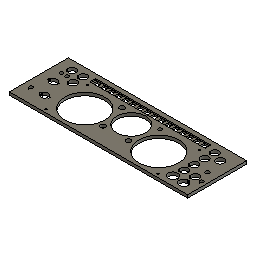
unimog dash old style (Autodesk Fusion 360 design; units mm, degrees)
part number: 2026-06-18-12-45-24-392
Autodesk Fusion 360 part; units mm, degrees
sketch "Sketch1" plane through (0, 0, 0) normal (0, 1, 0) x (1, 0, 0)
  line L0 (0, 0) -> (650, 0)
  line L1 (650, 0) -> (650, 215)
  line L2 (650, 215) -> (0, 215)
  line L3 (0, 215) -> (0, 0)
  circle A0 centre (47.25, 182) radius 14
  circle A1 centre (87.25, 182) radius 14
  circle A2 centre (36, 154.5) radius 6
  circle A3 centre (56, 154.5) radius 6
  circle A4 centre (87.25, 145) radius 14
  circle A5 centre (47.25, 113.3) radius 13.2
  circle A6 centre (75.25, 53.75) radius 13.2
  circle A7 centre (25.25, 53.75) radius 6.25
  circle A8 centre (121.1645, 163.2) radius 3.4
  circle A9 centre (25.0509, 44.2521) radius 1.25
  circle A10 centre (121.1645, 12.4) radius 3.4
  circle A11 centre (190.3639, 84.625) radius 72.625
  circle A12 centre (255.4078, 155.4015) radius 9
  circle A13 centre (325.3694, 119.25) radius 52.75
  circle A14 centre (392.7247, 157.0764) radius 6
  circle A15 centre (460.375, 84.625) radius 72.625
  circle A16 centre (278.8118, 62.6996) radius 9
  circle A17 centre (371.927, 62.6996) radius 9
  circle A18 centre (529.5743, 163.2) radius 3.4
  circle A19 centre (529.5743, 12.4) radius 3.4
  circle A20 centre (567.25, 182) radius 14
  circle A21 centre (567.25, 145) radius 14
  circle A22 centre (567.25, 108) radius 14
  circle A23 centre (567.25, 71) radius 14
  circle A24 centre (563.125, 33.275) radius 16.875
  circle A25 centre (607.25, 71) radius 14
  circle A26 centre (605.25, 30) radius 16
  circle A27 centre (633.75, 68.25) radius 6.25
  circle A28 centre (615.85, 107.15) radius 7.15
  circle A29 centre (602.5, 166.5) radius 14.5
  line L4 (567.25, 71) -> (567.25, 182) construction
  line L5 (567.25, 71) -> (607.25, 71) construction
  line L6 (529.5743, 12.4) -> (529.5743, 163.2) construction
  line L7 (594.9763, 67.5652) -> (603.8152, 58.7263) construction
  line L8 (607.25, 71) -> (597.3539, 61.1039) construction
  line L9 (607.25, 71) -> (621.2468, 71) construction
  line L10 (594.9763, 67.5652) -> (592.6482, 65.2371) construction
  line L11 (592.6482, 65.2371) -> (601.4871, 56.3982)
  line L12 (601.4871, 56.3982) -> (602.8112, 57.7223)
  line L13 (607.25, 71) -> (617.1495, 80.8995) construction
  line L14 (593.9723, 66.5612) -> (592.6482, 65.2371)
  line L15 (603.8152, 58.7263) -> (601.4871, 56.3982) construction
  line L16 (605.1938, 75.6264) -> (595.1802, 65.6128) construction
  line L17 (600.0149, 75.127) -> (608.8537, 66.2882) construction
  line L18 (608.8537, 66.2882) -> (601.6878, 59.1222) construction
  line L19 (592.8489, 67.9611) -> (601.6878, 59.1222)
  line L20 (600.0149, 75.127) -> (592.8489, 67.9611) construction
  line L21 (567.25, 71) -> (557.3505, 61.1005) construction
  line L22 (560.5418, 73.1307) -> (569.3807, 64.2918) construction
  line L23 (569.3807, 64.2918) -> (561.4871, 56.3982) construction
  line L24 (552.6482, 65.2371) -> (561.4871, 56.3982)
  line L25 (560.5418, 73.1307) -> (552.6482, 65.2371) construction
  line L26 (567.25, 108) -> (557.0677, 97.8177) construction
  line L27 (556.1832, 105.7721) -> (565.0221, 96.9332) construction
  line L28 (565.0221, 96.9332) -> (561.4871, 93.3982) construction
  line L29 (552.6482, 102.2371) -> (561.4871, 93.3982)
  line L30 (556.1832, 105.7721) -> (552.6482, 102.2371) construction
  line L31 (567.25, 145) -> (557.3539, 135.1039) construction
  line L32 (555.9409, 142.5297) -> (564.7797, 133.6909) construction
  line L33 (564.7797, 133.6909) -> (561.4871, 130.3982) construction
  line L34 (552.6482, 139.2371) -> (561.4871, 130.3982)
  line L35 (555.9409, 142.5297) -> (552.6482, 139.2371) construction
  line L36 (567.25, 182) -> (557.3505, 172.1005) construction
  line L37 (552.8238, 176.4127) -> (561.6627, 167.5738) construction
  line L38 (561.6627, 167.5738) -> (561.4871, 167.3982) construction
  line L39 (552.6482, 176.2371) -> (561.4871, 167.3982)
  line L40 (552.8238, 176.4127) -> (552.6482, 176.2371) construction
  line L41 (552.6482, 176.2371) -> (552.736, 176.3249)
  line L42 (552.736, 176.3249) -> (553.9723, 177.5612)
  line L43 (561.4871, 167.3982) -> (562.8112, 168.7223)
  line L44 (552.6482, 139.2371) -> (553.9723, 140.5612)
  line L45 (561.4871, 130.3982) -> (562.8112, 131.7223)
  line L46 (552.6482, 65.2371) -> (553.9723, 66.5612)
  line L47 (561.4871, 56.3982) -> (562.8112, 57.7223)
  line L48 (561.4871, 93.3982) -> (562.8112, 94.7223)
  line L49 (552.6482, 102.2371) -> (553.9723, 103.5612)
  line L50 (371.927, 62.6996) -> (278.8118, 62.6996) construction
  line L51 (460.375, 84.625) -> (190.3639, 84.625) construction
  line L52 (121.1645, 12.4) -> (529.5743, 12.4) construction
  line L53 (121.1645, 12.4) -> (121.1645, 163.2) construction
  line L54 (121.1645, 163.2) -> (529.5743, 163.2) construction
  line L55 (605.25, 14) -> (605.25, 30) construction
  line L56 (605.25, 30) -> (605.25, 46) construction
  line L57 (546.25, 33.275) -> (563.125, 33.275) construction
  line L58 (563.125, 33.275) -> (580, 33.275) construction
  line L59 (602, 48) -> (608.5, 48)
  line L60 (608.5, 48) -> (608.5, 43.3355)
  line L61 (608.5, 43.3355) -> (602, 43.3355)
  line L62 (602, 43.3355) -> (602, 48)
  line L63 (578.0171, 36.025) -> (580.75, 36.025)
  line L64 (580.75, 36.025) -> (580.75, 30.525)
  line L65 (580.75, 30.525) -> (578.0171, 30.525)
  line L66 (578.0171, 30.525) -> (578.0171, 36.025)
  circle A30 centre (633.75, 58.75) radius 1.25
  line L67 (633.75, 68.25) -> (633.75, 58.75) construction
  line L68 (87.25, 145) -> (77.3505, 135.1005) construction
  line L69 (87.25, 182) -> (77.3505, 172.1005) construction
  line L70 (47.25, 182) -> (37.3505, 172.1005) construction
  line L71 (87.25, 145) -> (87.25, 182) construction
  line L72 (87.25, 182) -> (47.25, 182) construction
  line L73 (36, 154.5) -> (56, 154.5) construction
  line L74 (567.25, 182) -> (87.25, 182) construction
  line L75 (557.3505, 61.1005) -> (557.0677, 60.8177) construction
  line L76 (557.3539, 135.1039) -> (550.2188, 127.9688) construction
  line L77 (32.3849, 176.5004) -> (41.2238, 167.6616)
  line L78 (32.3849, 176.5004) -> (33.8453, 177.9608)
  line L79 (41.2238, 167.6616) -> (42.4213, 168.8591)
  line L80 (87.25, 182) -> (76.9585, 171.7085) construction
  line L81 (72.6482, 176.2371) -> (74.0824, 177.2446)
  line L82 (81.4871, 167.3982) -> (82.8112, 168.7223)
  line L83 (87.25, 145) -> (77.0677, 134.8177) construction
  line L84 (72.6482, 139.2371) -> (73.9723, 140.5612)
  line L85 (72.6482, 139.2371) -> (81.4871, 130.3982)
  line L86 (81.4871, 130.3982) -> (82.8112, 131.7223)
  line L87 (72.6482, 176.2371) -> (81.4871, 167.3982)
  line L88 (76.9585, 171.7085) -> (77.0677, 171.8177) construction
  line L89 (30.5, 117.05) -> (64, 117.05)
  line L90 (64, 117.05) -> (64, 109.55)
  line L91 (64, 109.55) -> (30.5, 109.55)
  line L92 (30.5, 109.55) -> (30.5, 117.05)
  line L93 (47.25, 117.05) -> (47.25, 113.3) construction
  line L94 (47.25, 113.3) -> (30.5, 113.3) construction
  line L95 (92, 50) -> (58.5, 50)
  line L96 (75.25, 53.75) -> (58.5, 53.75) construction
  line L97 (75.25, 57.5) -> (75.25, 53.75) construction
  line L98 (58.5, 50) -> (58.5, 57.5)
  line L99 (58.5, 57.5) -> (92, 57.5)
  line L100 (92, 57.5) -> (92, 50)
  line L101 (47.25, 182) -> (47.25, 113.3) construction
  line L102 (75.25, 53.75) -> (25.25, 53.75) construction
  line L103 (115.3694, 199) -> (535.3694, 199)
  line L104 (535.3694, 199) -> (535.3694, 178.5)
  line L105 (535.3694, 178.5) -> (115.3694, 178.5)
  line L106 (115.3694, 178.5) -> (115.3694, 199)
  line L107 (325.3694, 119.25) -> (325.3694, 178.5) construction
  line L108 (122.3694, 198) -> (138.3694, 198)
  line L109 (138.3694, 198) -> (138.3694, 179.5)
  line L110 (138.3694, 179.5) -> (122.3694, 179.5)
  line L111 (122.3694, 179.5) -> (122.3694, 198)
  line L112 (115.3694, 188.75) -> (122.3694, 188.75)
  line L113 (148.3694, 179.5) -> (148.3694, 198)
  line L114 (148.3694, 198) -> (164.3694, 198)
  line L115 (164.3694, 198) -> (164.3694, 179.5)
  line L116 (164.3694, 179.5) -> (148.3694, 179.5)
  line L117 (174.3694, 179.5) -> (174.3694, 198)
  line L118 (174.3694, 198) -> (190.3694, 198)
  line L119 (190.3694, 198) -> (190.3694, 179.5)
  line L120 (190.3694, 179.5) -> (174.3694, 179.5)
  line L121 (200.3694, 179.5) -> (200.3694, 198)
  line L122 (200.3694, 198) -> (216.3694, 198)
  line L123 (216.3694, 198) -> (216.3694, 179.5)
  line L124 (216.3694, 179.5) -> (200.3694, 179.5)
  line L125 (226.3694, 179.5) -> (226.3694, 198)
  line L126 (226.3694, 198) -> (242.3694, 198)
  line L127 (242.3694, 198) -> (242.3694, 179.5)
  line L128 (242.3694, 179.5) -> (226.3694, 179.5)
  line L129 (252.3694, 179.5) -> (252.3694, 198)
  line L130 (252.3694, 198) -> (268.3694, 198)
  line L131 (268.3694, 198) -> (268.3694, 179.5)
  line L132 (268.3694, 179.5) -> (252.3694, 179.5)
  line L133 (278.3694, 179.5) -> (278.3694, 198)
  line L134 (278.3694, 198) -> (294.3694, 198)
  line L135 (294.3694, 198) -> (294.3694, 179.5)
  line L136 (294.3694, 179.5) -> (278.3694, 179.5)
  line L137 (304.3694, 179.5) -> (304.3694, 198)
  line L138 (304.3694, 198) -> (320.3694, 198)
  line L139 (320.3694, 198) -> (320.3694, 179.5)
  line L140 (320.3694, 179.5) -> (304.3694, 179.5)
  line L141 (330.3694, 179.5) -> (330.3694, 198)
  line L142 (330.3694, 198) -> (346.3694, 198)
  line L143 (346.3694, 198) -> (346.3694, 179.5)
  line L144 (346.3694, 179.5) -> (330.3694, 179.5)
  line L145 (356.3694, 179.5) -> (356.3694, 198)
  line L146 (356.3694, 198) -> (372.3694, 198)
  line L147 (372.3694, 198) -> (372.3694, 179.5)
  line L148 (372.3694, 179.5) -> (356.3694, 179.5)
  line L149 (382.3694, 179.5) -> (382.3694, 198)
  line L150 (382.3694, 198) -> (398.3694, 198)
  line L151 (398.3694, 198) -> (398.3694, 179.5)
  line L152 (398.3694, 179.5) -> (382.3694, 179.5)
  line L153 (408.3694, 179.5) -> (408.3694, 198)
  line L154 (408.3694, 198) -> (424.3694, 198)
  line L155 (424.3694, 198) -> (424.3694, 179.5)
  line L156 (424.3694, 179.5) -> (408.3694, 179.5)
  line L157 (434.3694, 179.5) -> (434.3694, 198)
  line L158 (434.3694, 198) -> (450.3694, 198)
  line L159 (450.3694, 198) -> (450.3694, 179.5)
  line L160 (450.3694, 179.5) -> (434.3694, 179.5)
  line L161 (460.3694, 179.5) -> (460.3694, 198)
  line L162 (460.3694, 198) -> (476.3694, 198)
  line L163 (476.3694, 198) -> (476.3694, 179.5)
  line L164 (476.3694, 179.5) -> (460.3694, 179.5)
  line L165 (486.3694, 179.5) -> (486.3694, 198)
  line L166 (486.3694, 198) -> (502.3694, 198)
  line L167 (502.3694, 198) -> (502.3694, 179.5)
  line L168 (502.3694, 179.5) -> (486.3694, 179.5)
  line L169 (512.3694, 179.5) -> (512.3694, 198)
  line L170 (512.3694, 198) -> (528.3694, 198)
  line L171 (528.3694, 198) -> (528.3694, 179.5)
  line L172 (528.3694, 179.5) -> (512.3694, 179.5)
  point P0 (599.3958, 63.1458)
  point P1 (605.25, 43.3355)
  point P2 (578.0171, 33.275)
  point P3 (557.0677, 60.8177)
  point P4 (557.0677, 134.8177)
  point P5 (557.0677, 97.8177)
  point P6 (77.3505, 172.1005)
  point P7 (77.0677, 134.8177)
  point P8 (77.0677, 171.8177)
  point P9 (75.25, 57.5)
  point P10 (325.3694, 178.5)
  dimension "d1" = 650
  dimension "d2" = 215
  dimension "d3" = 32
  dimension "d4" = 14
  dimension "d5" = 28.75
  dimension "d6" = 12.5
  dimension "d7" = 10
  dimension "d8" = 62
  dimension "d9" = 28
  dimension "d10" = 28
  dimension "d11" = 28
  dimension "d12" = 28
  dimension "d13" = 28
  dimension "d14" = 33.75
  dimension "d15" = 16.4
  dimension "d16" = 70
  dimension "d17" = 6.8
  dimension "d19" = 9
  dimension "d20" = 28.75
  dimension "d21" = 57
  dimension "d22" = 12
  dimension "d23" = 9
  dimension "d24" = 9
  dimension "d25" = 9
  dimension "d26" = 19
  dimension "d27" = 29
  dimension "d28" = 33
  dimension "d29" = 34
  dimension "d30" = 14.3
  dimension "d31" = 27
  dimension "d32" = 100
  dimension "d33" = 6.8
  dimension "d34" = 144
  dimension "d35" = 145.25
  dimension "d36" = 145.25
  dimension "d37" = 12
  dimension "d38" = 117
  dimension "d39" = 12.5
  dimension "d40" = 135
  dimension "d41" = 28.4
  dimension "d42" = 12.5
  dimension "d43" = 12.5
  dimension "d44" = 12.5
  dimension "d45" = 12.5
  dimension "d46" = 12.5
  dimension "d47" = 66.5
  dimension "d48" = 105.5
  dimension "d49" = 14
  dimension "d50" = 12
  dimension "d51" = 18
  dimension "d52" = 18
  dimension "d53" = 18
  dimension "d54" = 9.5
  dimension "d55" = 11.5
  dimension "d56" = 11.5
  dimension "d57" = 9.5
  dimension "d58" = 14
  dimension "d59" = 6.8
  dimension "d62" = 24
  dimension "d63" = 408.4098
  dimension "d64" = 24
  dimension "d65" = 20.5
  dimension "d66" = 18.5
  dimension "d67" = 17
  dimension "d70" = 14.5
  dimension "d71" = 6.8
  dimension "d74" = 6.5
  dimension "d75" = 34
  dimension "d76" = 5.5
  dimension "d77" = 34.5
  dimension "d78" = 2.5
  dimension "d79" = 2
  dimension "d80" = 28
  dimension "d81" = 28
  dimension "d82" = 28
  dimension "d83" = 12
  dimension "d84" = 12
  dimension "d85" = 2.5
  dimension "d86" = 2
  dimension "d87" = 12.5
  dimension "d88" = 19
  dimension "d89" = 47.5
  dimension "d90" = 12
  dimension "d91" = 9
  dimension "d92" = 33.25
  dimension "d93" = 30
  dimension "d94" = 54.5
  dimension "d95" = 8
  dimension "d96" = 28.4
  dimension "d98" = 28.4
  dimension "d99" = 28.4
  dimension "d100" = 12.5
  dimension "d101" = 28.4
  dimension "d102" = 12.5
  dimension "d103" = 12.5
  dimension "d104" = 28.4
  dimension "d105" = 28.4
  dimension "d106" = 26.4
  dimension "d107" = 26.4
  dimension "d108" = 33.5
  dimension "d110" = 33.5
  dimension "d112" = 7.5
  dimension "d113" = 3.75
  dimension "d114" = 27
  dimension "d115" = 41.5
  dimension "d116" = 20.5
  dimension "d117" = 420
  dimension "d118" = 6.5
  dimension "d119" = 16
  dimension "d120" = 18.5
  dimension "d121" = 7
  dimension "d124" = 26
  dimension "d125" = 0
  dimension "d126" = 7
  constraint horizontal L0
  constraint vertical L1
  constraint horizontal L2
  constraint vertical L3
  constraint coincident L0.start L3.end
  constraint coincident A23.centre L4.start
  constraint coincident A20.centre L4.end
  constraint coincident A21.centre L4
  constraint coincident A22.centre L4
  constraint vertical L4
  constraint coincident A25.centre L5.end
  constraint horizontal L5
  constraint coincident A19.centre L6.start
  constraint coincident A18.centre L6.end
  constraint vertical L6
  constraint horizontal L9
  constraint perpendicular L7 L8
  constraint midpoint L7 P0
  constraint coincident L8 P0
  constraint perpendicular L7 L10
  constraint perpendicular L10 L11
  constraint parallel L10 L12
  constraint collinear L8 L13
  constraint coincident A25 L13.end
  constraint coincident A25 L14.start
  constraint coincident L10 L14.start
  constraint perpendicular L11 L14
  constraint coincident A25 L12.end
  constraint perpendicular L11 L15
  constraint perpendicular L16 L17
  constraint perpendicular L17 L20
  constraint perpendicular L19 L20
  constraint perpendicular L18 L19
  constraint perpendicular L21 L22
  constraint perpendicular L22 L25
  constraint perpendicular L24 L25
  constraint perpendicular L23 L24
  constraint perpendicular L26 L27
  constraint perpendicular L27 L30
  constraint perpendicular L29 L30
  constraint perpendicular L28 L29
  constraint perpendicular L31 L32
  constraint perpendicular L32 L35
  constraint perpendicular L34 L35
  constraint perpendicular L33 L34
  constraint perpendicular L36 L37
  constraint perpendicular L37 L40
  constraint perpendicular L39 L40
  constraint perpendicular L38 L39
  constraint midpoint L40 L41.end
  constraint coincident A20 L42.end
  constraint coincident L40 L42.end
  constraint coincident A20 L43.end
  constraint coincident L38 L43.end
  constraint coincident L35 L44.end
  constraint coincident A21 L44.end
  constraint coincident A21 L45.end
  constraint coincident L33 L45.end
  constraint coincident A23 L46.end
  constraint coincident L25 L46.end
  constraint coincident L23 L47.end
  constraint coincident A23 L47.end
  constraint coincident A22 L48.end
  constraint coincident L28 L48.end
  constraint coincident L30 L49.end
  constraint coincident A22 L49.end
  constraint coincident A17.centre L50.start
  constraint coincident A16.centre L50.end
  constraint horizontal L50
  constraint coincident A15.centre L51.start
  constraint coincident A11.centre L51.end
  constraint horizontal L51
  constraint coincident A10.centre L52.start
  constraint horizontal L52
  constraint coincident A8.centre L53.end
  constraint vertical L53
  constraint horizontal L54
  constraint coincident A26 L55.start
  constraint coincident A26.centre L55.end
  constraint coincident A26 L56.end
  constraint perpendicular L0 L56
  constraint collinear L55 L56
  constraint coincident A24 L57.start
  constraint coincident A24.centre L57.end
  constraint coincident A24 L58.end
  constraint parallel L57 L58
  constraint horizontal L58
  constraint horizontal L59
  constraint vertical L60
  constraint horizontal L61
  constraint vertical L62
  constraint midpoint L61 P1
  constraint coincident L56 P1
  constraint horizontal L63
  constraint vertical L64
  constraint horizontal L65
  constraint vertical L66
  constraint midpoint L66 P2
  constraint coincident L58 P2
  constraint coincident A27.centre L67.start
  constraint coincident A30.centre L67.end
  constraint vertical L67
  constraint coincident A4.centre L68.start
  constraint coincident A1.centre L69.start
  constraint coincident L70 A0.centre
  constraint horizontal L72
  constraint vertical L71
  constraint coincident A0.centre L70.start
  constraint coincident A2.centre L73.start
  constraint coincident A3.centre L73.end
  constraint horizontal L73
  constraint horizontal L74
  constraint coincident A23 L21.end
  constraint midpoint L24 P3
  constraint coincident P3 L75.end
  constraint perpendicular L24 L75
  constraint parallel L16 L21
  constraint parallel L8 L16
  constraint parallel L21 L26
  constraint parallel L26 L31
  constraint coincident A20 L36.end
  constraint perpendicular L32 L76
  constraint coincident A21.centre L31.start
  constraint midpoint L34 P4
  constraint coincident L76 P4
  constraint coincident A22.centre L26.start
  constraint coincident P5 L29
  constraint midpoint L29 P5
  constraint coincident P5 L26.end
  constraint coincident A1 P6
  constraint coincident A0 L70.end
  constraint coincident A4 L68.end
  constraint perpendicular L70 L77
  constraint coincident A0 L78.end
  constraint perpendicular L77 L78
  constraint coincident A0 L79.end
  constraint perpendicular L77 L79
  constraint coincident P6 L69.end
  constraint collinear L69 L80
  constraint coincident A1 L82.end
  constraint coincident A1 L81.end
  constraint perpendicular L83 L85
  constraint perpendicular L84 L85
  constraint perpendicular L85 L86
  constraint coincident P7 L85
  constraint parallel L68 L69
  constraint parallel L68 L83
  constraint midpoint L85 P7
  constraint coincident P7 L83.end
  constraint coincident A4 L84.end
  constraint coincident A4 L86.end
  constraint perpendicular L82 L87
  constraint midpoint L87 P8
  constraint parallel L69 L88
  constraint coincident P8 L88.end
  constraint parallel L70 L80
  constraint parallel L77 L87
  constraint horizontal L89
  constraint vertical L90
  constraint horizontal L91
  constraint vertical L92
  constraint midpoint L89 L93.start
  constraint coincident A5.centre L93.end
  constraint vertical L93
  constraint midpoint L92 L94.end
  constraint horizontal L94
  constraint vertical L100
  constraint horizontal L95
  constraint vertical L98
  constraint vertical L97
  constraint midpoint L96.end L98
  constraint horizontal L96
  constraint horizontal L99
  constraint coincident A6.centre L96.start
  constraint vertical L101
  constraint midpoint L99 P9
  constraint coincident P9 L97.start
  constraint coincident L98.end L99.start
  constraint coincident L99.end L100.start
  constraint coincident A7.centre L102.end
  constraint horizontal L102
  constraint horizontal L103
  constraint vertical L104
  constraint horizontal L105
  constraint vertical L106
  constraint midpoint L105 P10
  constraint coincident A13.centre L107.start
  constraint coincident P10 L107.end
  constraint vertical L107
  constraint horizontal L108
  constraint vertical L109
  constraint horizontal L110
  constraint vertical L111
  constraint midpoint L106 L112.start
  constraint midpoint L111 L112.end
  constraint horizontal L112
  measures "d1" distance of L0.start L0.end
  measures "d2" distance of L0.end L1.end
  measures "d3" diameter of A26
  measures "d4" distance of L0 A26
  measures "d5" distance of L1 A26
  measures "d6" diameter of A27
  measures "d7" distance of L1 A27
  measures "d8" distance of L0 A27
  measures "d9" diameter of A25
  measures "d10" diameter of A23
  measures "d11" diameter of A22
  measures "d12" diameter of A21
  measures "d13" diameter of A20
  measures "d14" diameter of A24
  measures "d15" distance of L0 A24
  measures "d16" distance of L1 A24
  measures "d17" diameter of A19
  measures "d19" distance of L0 A19
  measures "d20" distance of L1 A25
  measures "d21" distance of L0 A25
  measures "d22" distance of A23 A25
  measures "d23" distance of A22 A23
  measures "d24" distance of A21 A22
  measures "d25" distance of A20 A21
  measures "d26" distance of L2 A20
  measures "d27" diameter of A29
  measures "d28" distance of L1 A29
  measures "d29" distance of L2 A29
  measures "d30" diameter of A28
  measures "d31" distance of L1 A28
  measures "d32" distance of L0 A28
  measures "d33" diameter of A18
  measures "d34" distance of A18 A19
  measures "d35" diameter of A15
  measures "d36" diameter of A11
  measures "d37" distance of L0 A15
  measures "d38" distance of L1 A15
  measures "d39" distance of L7.start L7.end
  measures "d40" angle of L8 L9
  measures "d41" distance of L11 L13.end
  measures "d42" distance of L17.end L17.start
  measures "d43" distance of L22.end L22.start
  measures "d44" distance of L27.end L27.start
  measures "d45" distance of L32.end L32.start
  measures "d46" distance of L37.end L37.start
  measures "d47" distance of L0 A13
  measures "d48" diameter of A13
  measures "d49" distance of A13 A15
  measures "d50" diameter of A14
  measures "d51" diameter of A12
  measures "d52" diameter of A16
  measures "d53" diameter of A17
  measures "d54" distance of A15 A17
  measures "d55" distance of A13 A17
  measures "d56" distance of A13 A16
  measures "d57" distance of A11 A16
  measures "d58" distance of A11 A13
  measures "d59" diameter of A10
  measures "d62" distance of A10 A11
  measures "d63" distance of A10.centre A19.centre
  measures "d64" distance of A15 A19
  measures "d65" distance of A14 A15
  measures "d66" distance of A13 A14
  measures "d67" distance of A12 A13
  measures "d70" distance of A11 A12
  measures "d71" diameter of A8
  measures "d74" distance of L59.start L59.end
  measures "d75" distance of L55.start L59
  measures "d76" distance of L63.end L64.end
  measures "d77" distance of L57.start L64
  measures "d78" diameter of A30
  measures "d79" distance of A27 A30
  measures "d80" diameter of A4
  measures "d81" diameter of A1
  measures "d82" diameter of A0
  measures "d83" diameter of A3
  measures "d84" diameter of A2
  measures "d85" diameter of A9
  measures "d86" distance of A7 A9
  measures "d87" diameter of A7
  measures "d88" distance of L3 A7
  measures "d89" distance of L0 A7
  measures "d90" distance of A0 A1
  measures "d91" distance of A1 A4
  measures "d92" distance of L3 A0
  measures "d93" distance of L3 A2
  measures "d94" distance of L2 A2
  measures "d95" distance of A2 A3
  measures "d100" distance of L77.start L77.end
  measures "d102" distance of L81.start L82.start
  measures "d103" distance of L84.start L85.end
  measures "d106" diameter of A5
  measures "d107" diameter of A6
  measures "d108" distance of L90 L92
  measures "d110" distance of L98 L100
  measures "d112" distance of L89 L91
  measures "d113" distance of A6.centre P9
  measures "d114" distance of A7 L96.end
  measures "d115" distance of A0 A5
  measures "d116" distance of L103 L105
  measures "d117" distance of L103.start L103.end
  measures "d118" distance of A13 L105
  measures "d119" distance of L108.start L108.end
  measures "d120" distance of L108.start L110.end
  measures "d121" distance of L106 L111
  measures "d126" distance of L104 L171
extrude "Extrude1" add sketch "Sketch1" against normal blind 11 contours L0 L1 L2 L3 | L103 L104 L105 L106 | L108 L109 L110 L111 | L113 L114 L115 L116 | L117 L118 L119 L120 | L121 L122 L123 L124 | L125 L126 L127 L128 | L129 L130 L131 L132 | L133 L134 L135 L136 | L137 L138 L139 L140 | L141 L142 L143 L144 | L145 L146 L147 L148 | L149 L150 L151 L152 | L153 L154 L155 L156 | L157 L158 L159 L160 | L161 L162 L163 L164 | L165 L166 L167 L168 | L169 L170 L171 L172
extrude "Extrude2" cut sketch "Sketch1" against normal blind 4.5 contours L103 L104 L105 L106
extrude "Extrude3" cut sketch "Sketch1" against normal blind 140 contours L108 L109 L110 L111 | L113 L114 L115 L116 | L117 L118 L119 L120 | L121 L122 L123 L124 | L125 L126 L127 L128 | L129 L130 L131 L132 | L133 L134 L135 L136 | L137 L138 L139 L140 | L141 L142 L143 L144 | L145 L146 L147 L148 | L149 L150 L151 L152 | L153 L154 L155 L156 | L157 L158 L159 L160 | L161 L162 L163 L164 | L165 L166 L167 L168 | L169 L170 L171 L172
equation "d33 = d17"
equation "d36 = d35"
equation "d59 = d17"
equation "d71 = d59"
equation "d113 = ( 7.5 / 2 ) * 1 mm"
